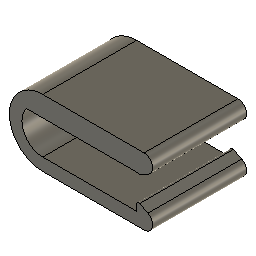
z_belt_clip (Autodesk Fusion 360 design; units mm, degrees)
Autodesk Fusion 360 part; units mm, degrees
note: some values were not read from the file. Chosen so that the rebuilt part matches the saved one: where a step ends.
sketch "Sketch1" plane through (0, 0, 0) normal (0, 1, 0) x (1, 0, 0)
  line L0 (0, 2) -> (9, 2)
  line L1 (0, -2) -> (9, -2)
  arc A0 (0, 2) -> (0, -2) centre (0, 0) ccw
  line L2 (9, 2) -> (9, 1.4)
  line L3 (9.2894, 1.2211) -> (10.0894, 1.6211)
  line L4 (10, 2) -> (9, 2)
  arc A1 (10.0894, 1.6211) -> (10, 2) centre (10, 1.8) ccw
  arc A2 (9, 1.4) -> (9.2894, 1.2211) centre (9.2, 1.4) ccw
  line L5 (0, 3.2) -> (9.7167, 3.2)
  arc A3 (10.0894, 1.6211) -> (9.7167, 3.2) centre (9.7167, 2.3666) ccw
  arc A4 (0, 3.2) -> (0, -3.2) centre (0, 0) ccw
  line L6 (0, -3.2) -> (9.8114, -3.2)
  line L7 (9.2, 1.2) -> (-1.6, 1.2)
  line L8 (-1.6363, 1.15) -> (9.5735, 1.15) construction
  arc A5 (0.5915, 1.2804) -> (0.4989, 1.5882) centre (-0.4, 1.15) ccw
  arc A6 (0.4989, 1.5882) -> (-0.5512, 1.2804) centre (0, 1.345) ccw
  line L9 (0.5915, 1.2804) -> (3.8872, 1.2804) construction
  arc A7 (0.5915, 1.2804) -> (0.7402, 1.15) centre (0.7402, 1.3) ccw
  line L10 (0.5915, 1.2804) -> (-1.1534, 1.2804) construction
  line L11 (0, 1.345) -> (2.0709, 1.345) construction
  line L12 (0.7402, 1.15) -> (1.3137, 1.15)
  arc A8 (1.3137, 1.15) -> (1.4034, 1.2326) centre (1.3137, 1.24) ccw
  arc A9 (1.5011, 1.5882) -> (1.4034, 1.2326) centre (2.4, 1.15) ccw
  arc A10 (2.5512, 1.2804) -> (1.5011, 1.5882) centre (2, 1.345) ccw
  line L13 (0, 1.345) -> (0, 1.7795) construction
  arc A11 (2.6506, 1.2688) -> (1.4112, 1.632) centre (2, 1.345) ccw
  arc A12 (1.4112, 1.632) -> (1.3046, 1.25) centre (2.4, 1.15) ccw
  line L14 (0.7402, 1.25) -> (1.3046, 1.25)
  arc A13 (0.6906, 1.2935) -> (0.7402, 1.25) centre (0.7402, 1.3) ccw
  arc A14 (0.6906, 1.2935) -> (0.5888, 1.632) centre (-0.4, 1.15) ccw
  arc A15 (0.5888, 1.632) -> (-0.6506, 1.2688) centre (0, 1.345) ccw
  line L15 (1.75, 0) -> (22.5, 0)
  line L16 (9, -2) -> (9, -1.4)
  arc A16 (9.2894, -1.2211) -> (9, -1.4) centre (9.2, -1.4) ccw
  line L17 (9.2894, -1.2211) -> (10.0894, -1.6211)
  arc A17 (9.7167, -3.2) -> (10.0894, -1.6211) centre (9.7167, -2.3666) ccw
  arc A18 (10, -2) -> (10.0894, -1.6211) centre (10, -1.8) ccw
  line L18 (10, -2) -> (9, -2)
  dimension "d1" = 4
  dimension "d2" = 9
  dimension "d4" = 0.4
  dimension "d5" = 1
  dimension "d8" = 0.6
  dimension "d10" = 1.2
  dimension "d17" = 1.11
  dimension "d18" = 2
  dimension "d19" = 0.195
  dimension "d20" = 0.3
  dimension "d21" = 2
  dimension "d22" = 0.1
  dimension "d23" = 0.1
  constraint coincident A0.centre A4.centre
  constraint horizontal L0
  constraint horizontal L1
  constraint tangent L0 A0
  constraint tangent L1 A0
  constraint equal L0 L1
  constraint perpendicular L0 L2
  constraint tangent L4 A1
  constraint tangent L3 A1
  constraint collinear L0 L4
  constraint tangent L2 A2
  constraint tangent L3 A2
  constraint equal A1 A2
  constraint horizontal L5
  constraint tangent L5 A3
  constraint tangent L3 A3
  constraint tangent L5 A4
  constraint horizontal L6
  constraint tangent A4 L6
  constraint coincident A0 L7.end
  constraint horizontal L7
  constraint tangent A2 L7
  constraint coincident A2 L7.start
  constraint tangent A5 A6
  constraint horizontal L8
  constraint coincident A5.centre L8
  constraint tangent L8 A7
  constraint tangent A5 A7
  constraint coincident A0 L8.start
  constraint parallel L8 L9
  constraint parallel L9 L10
  constraint coincident L10 A6.end
  constraint coincident A6.centre L11.start
  constraint parallel L0 L11
  constraint coincident A10.centre L11
  constraint equal A6 A10
  constraint equal A5 A9
  constraint coincident L8 A9.centre
  constraint tangent A9 A10
  constraint tangent L8 A8
  constraint tangent A8 A9
  constraint coincident L8 A7.end
  constraint coincident L8 L12.end
  constraint coincident L9 A10.start
  constraint vertical L13
  constraint coincident L0.start L13
  constraint symmetric L0.end L15 L1.end
  constraint symmetric L3.end L15 L17.end
  constraint symmetric L4.start L15 A18.start
  constraint symmetric L2.end L15 L16.end
  constraint symmetric L3.start L15 A16.start
  constraint symmetric A1 L15 A18
  constraint symmetric A2 L15 A16
  constraint symmetric L5.end L15 A17.start
  constraint symmetric A3 L15 A17
  measures "d1" diameter of A0
  measures "d2" distance of L0.end L0.start
  measures "d4" diameter of A1
  measures "d5" distance of L0.end L4.start
  measures "d8" vertical distance of L0.end A2.centre
  measures "d10" distance of L0 L5
  measures "d17" diameter of A6
  measures "d18" diameter of A5
  measures "d19" vertical distance of A6.centre A5.centre
  measures "d20" diameter of A7
  measures "d21" distance of A6.centre A10.centre
  measures "d22" distance of L0 A6
extrude "Extrude1" add sketch "Sketch1" along normal blind 9 contours L0 L1 A0 L4 A1 L5 A3 A4 L6 A17 A18 L18 | L2 L3 L4 A1 A2 | L16 A16 L17 A18 L18
sketch "Sketch2" plane through (0, 0, 0) normal (1, 0, 0) x (0, 1, 0)
  line L0 (0, 2) -> (9, 2)
  line L1 (9.3429, 1.15) -> (-3.2287, 1.15) construction
  arc A0 (0.2598, 1.15) -> (0.4085, 1.2804) centre (0.2598, 1.3) ccw
  arc A1 (0.5011, 1.5882) -> (0.4085, 1.2804) centre (1.4, 1.15) ccw
  arc A2 (1.4989, 1.5882) -> (0.5011, 1.5882) centre (1, 1.345) ccw
  arc A3 (1.5915, 1.2804) -> (1.4989, 1.5882) centre (0.6, 1.15) ccw
  arc A4 (1.5915, 1.2804) -> (1.7402, 1.15) centre (1.7402, 1.3) ccw
  arc A5 (0.2598, 1.25) -> (0.3094, 1.2935) centre (0.2598, 1.3) ccw
  arc A6 (0.4112, 1.632) -> (0.3094, 1.2935) centre (1.4, 1.15) ccw
  arc A7 (1.5888, 1.632) -> (0.4112, 1.632) centre (1, 1.345) ccw
  arc A8 (1.6906, 1.2935) -> (1.5888, 1.632) centre (0.6, 1.15) ccw
  arc A9 (1.6906, 1.2935) -> (1.7402, 1.25) centre (1.7402, 1.3) ccw
  line L2 (0.2598, 1.25) -> (0, 1.25)
  line L3 (1.7402, 1.25) -> (2, 1.25)
  line L4 (2, 1.25) -> (2, 2)
  line L5 (0, 2) -> (0, 1.25)
  line L6 (2.2598, 1.25) -> (2, 1.25)
  arc A10 (2.2598, 1.25) -> (2.3094, 1.2935) centre (2.2598, 1.3) ccw
  arc A11 (2.4112, 1.632) -> (2.3094, 1.2935) centre (3.4, 1.15) ccw
  arc A12 (3.5888, 1.632) -> (2.4112, 1.632) centre (3, 1.345) ccw
  arc A13 (3.6906, 1.2935) -> (3.5888, 1.632) centre (2.6, 1.15) ccw
  arc A14 (3.6906, 1.2935) -> (3.7402, 1.25) centre (3.7402, 1.3) ccw
  line L7 (3.7402, 1.25) -> (4, 1.25)
  line L8 (4, 1.25) -> (4, 2)
  line L9 (4.2598, 1.25) -> (4, 1.25)
  arc A15 (4.2598, 1.25) -> (4.3094, 1.2935) centre (4.2598, 1.3) ccw
  arc A16 (4.4112, 1.632) -> (4.3094, 1.2935) centre (5.4, 1.15) ccw
  arc A17 (5.5888, 1.632) -> (4.4112, 1.632) centre (5, 1.345) ccw
  arc A18 (5.6906, 1.2935) -> (5.5888, 1.632) centre (4.6, 1.15) ccw
  arc A19 (5.6906, 1.2935) -> (5.7402, 1.25) centre (5.7402, 1.3) ccw
  line L10 (5.7402, 1.25) -> (6, 1.25)
  line L11 (6, 1.25) -> (6, 2)
  line L12 (6.2598, 1.25) -> (6, 1.25)
  arc A20 (6.2598, 1.25) -> (6.3094, 1.2935) centre (6.2598, 1.3) ccw
  arc A21 (6.4112, 1.632) -> (6.3094, 1.2935) centre (7.4, 1.15) ccw
  arc A22 (7.5888, 1.632) -> (6.4112, 1.632) centre (7, 1.345) ccw
  arc A23 (7.6906, 1.2935) -> (7.5888, 1.632) centre (6.6, 1.15) ccw
  arc A24 (7.6906, 1.2935) -> (7.7402, 1.25) centre (7.7402, 1.3) ccw
  line L13 (7.7402, 1.25) -> (8, 1.25)
  line L14 (8, 1.25) -> (8, 2)
  line L15 (8.2598, 1.25) -> (8, 1.25)
  arc A25 (8.2598, 1.25) -> (8.3094, 1.2935) centre (8.2598, 1.3) ccw
  arc A26 (8.4112, 1.632) -> (8.3094, 1.2935) centre (9.4, 1.15) ccw
  arc A27 (9.5888, 1.632) -> (8.4112, 1.632) centre (9, 1.345) ccw
  arc A28 (9.6906, 1.2935) -> (9.5888, 1.632) centre (8.6, 1.15) ccw
  arc A29 (9.6906, 1.2935) -> (9.7402, 1.25) centre (9.7402, 1.3) ccw
  line L16 (9.7402, 1.25) -> (10, 1.25)
  line L17 (10, 1.25) -> (10, 2)
  dimension "d34" = 1.11
  dimension "d37" = 0.195
  dimension "d38" = 0.1
  dimension "d39" = 0.3
  dimension "d41" = 1
  dimension "d42" = 0.1
  dimension "d43" = 0.7402
  dimension "d47" = 1
  dimension "d48" = 1
  dimension "d51" = 2
  dimension "d52" = 0
  constraint tangent A1 A2
  constraint horizontal L1
  constraint coincident A1.centre L1
  constraint tangent L1 A0
  constraint tangent A0 A1
  constraint coincident L1 A0.start
  constraint coincident L1 A3.centre
  constraint tangent A2 A3
  constraint equal A1 A3
  constraint equal A0 A4
  constraint tangent L1 A4
  constraint tangent A3 A4
  constraint coincident L1 A4.end
  constraint tangent A5 L2
  constraint parallel L1 L2
  constraint tangent A9 L3
  constraint parallel L1 L3
  constraint coincident L0 L4.end
  constraint perpendicular L0 L4
  constraint coincident L0.start L5.start
  constraint perpendicular L2 L5
  measures "d34" diameter of A2
  measures "d37" distance of A2.centre L1
  measures "d38" distance of L0 A2
  measures "d39" diameter of A0
  measures "d41" radius of A1
  measures "d43" horizontal distance of A2.centre A9.end
  measures "d47" distance of A2.centre L4
  measures "d48" distance of A2.centre L5
extrude "Extrude3" add sketch "Sketch2" along normal up to far side of body 1 and the other way up to far side of body 1
equation "d17 = ( 0.555 * 2 ) * 1 mm"
equation "d19 = 0.75 mm - 0.555 mm"
equation "d34 = ( 0.555 * 2 ) * 1 mm"
equation "d37 = 0.75 mm - 0.555 mm"
equation "d48 = d47"
